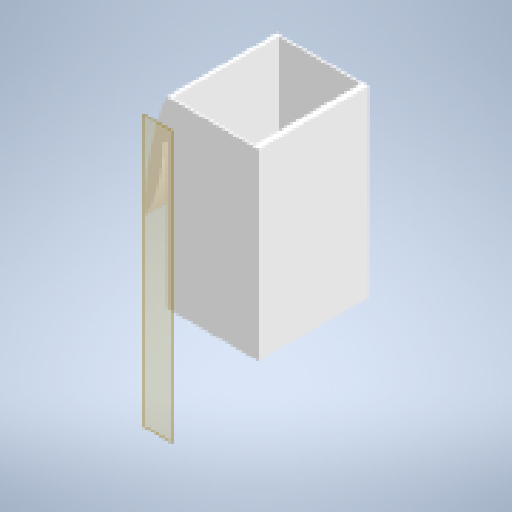
# Autodesk Inventor part: WingBox
Saved by Autodesk Inventor 2026 (Build 300175050, 175E)
## iProperties
Created: 2025-08-01
Part Number: WingBox
Material: Plastic, Opaque White
Document SubType Name: Modeling
Designer: Cupri
Mass: 728.648 g
Surface Area: 2482.51 cm^2
Volume: 765.387 cm^3
Density: 0.952 g/cm^3
Appearance: Smooth - White
Author: Cupri
Autodesk Inventor part; units mm, degrees
ref_plane "YZ Plane" through (0, 0, 0) normal (1, 0, 0) x (0, 1, 0)
ref_plane "XZ Plane" through (0, 0, 0) normal (0, 1, 0) x (-1, 0, 0)
ref_plane "XY Plane" through (0, 0, 0) normal (0, 0, 1) x (1, 0, 0)
ref_plane "Work Plane1" through (0, 0, 0) normal (0, 0, 1) x (1, 0, 0)
sketch "Sketch1" plane through (0, 0, 0) normal (0, 0, 1) x (1, 0, 0)
  line L0 (17.543857, 167.377737) -> (17.543857, -167.217661)
  line L1 (12.619782, 167.377737) -> (17.543857, 167.377737)
  arc A0 (12.619782, 167.377737) -> (7.619799, 162.364672) centre (12.619782, 162.377737) ccw
  arc A1 (-17.220572, 65.305302) -> (7.619799, 162.364672) centre (-192.379519, 161.842048) ccw
  spline S0 degree 3 poles (15.506608, -167.377737) (14.147951, -162.345779) (13.145398, -158.732995) (12.220923, -155.352167) (11.293739, -151.961434) (10.445107, -148.803984) (9.518675, -145.1939) (8.592185, -141.583591) (7.587911, -137.520736) (6.471828, -132.825116) (5.346807, -128.091892) (4.10798, -122.714929) (2.846807, -117.031098) (1.553707, -111.203383) (0.259478, -105.140337) (-0.92675, -99.276727) (-2.132162, -93.318284) (-3.225902, -87.566367) (-4.23784, -81.945311) (-5.5682, -74.555504) (-6.790359, -67.285613) (-7.971575, -59.836625) (-9.552302, -49.86823) (-11.026112, -39.596979) (-12.264211, -29.351416) (-13.140881, -22.09676) (-13.908596, -14.883997) (-14.596958, -7.852484) (-15.268141, -0.996451) (-15.867695, 5.674384) (-16.352254, 12.543674) (-16.713746, 17.668333) (-17.004603, 22.971721) (-17.201941, 28.510361) (-17.39909, 34.043661) (-17.502934, 39.811858) (-17.52457, 45.347495) (-17.543857, 50.282258) (-17.501315, 54.954248) (-17.410102, 59.083092) (-17.361094, 61.301547) (-17.298032, 63.363057) (-17.220572, 65.305302) knots 0 0 0 0 0.06599902 0.06599902 0.06599902 0.13219142 0.13219142 0.13219142 0.19838797 0.19838797 0.19838797 0.26511464 0.26511464 0.26511464 0.33353047 0.33353047 0.33353047 0.40305279 0.40305279 0.40305279 0.49445138 0.49445138 0.49445138 0.61676292 0.61676292 0.61676292 0.70336901 0.70336901 0.70336901 0.78781372 0.78781372 0.78781372 0.85081155 0.85081155 0.85081155 0.91374865 0.91374865 0.91374865 0.96985415 0.96985415 0.96985415 1 1 1 1
  line L2 (16.076195, -167.223946) -> (15.506608, -167.377737)
  line L3 (17.264865, -167.218855) -> (16.076195, -167.223946)
  line L4 (17.26486, -167.217661) -> (17.264865, -167.218855)
  line L5 (17.543857, -167.217661) -> (17.26486, -167.217661)
  line L6 (-7.380943, 65.327391) -> (-7.294185, 45.068724)
  line L7 (12.904649, 65.39642) -> (-7.380943, 65.327391)
  line L8 (12.973526, 45.15552) -> (12.904649, 65.39642)
  line L9 (-7.294185, 45.068724) -> (12.973526, 45.15552)
  arc A2 (12.543857, 221.029621) -> (-17.220572, 65.305302) centre (332.504822, 79.16708) ccw
  line L10 (12.543857, 221.029621) -> (17.543857, 221.029621)
  line L11 (17.543857, 221.029621) -> (17.543857, 167.377737)
  line L12 (17.543857, 167.377737) -> (12.619782, 167.377737)
  arc A3 (12.619782, 167.577737) -> (7.419799, 162.364149) centre (12.619782, 162.377737) ccw
  line L13 (12.619782, 167.577737) -> (17.743857, 167.577737)
  line L14 (17.743857, 167.577737) -> (17.743857, -167.417661)
  line L15 (17.743857, -167.417661) -> (17.544285, -167.417661)
  line L16 (17.544285, -167.417661) -> (16.103141, -167.423832)
  line L17 (16.103141, -167.423832) -> (15.365657, -167.622957)
  arc A4 (-17.41853, 65.360482) -> (7.419799, 162.364149) centre (-192.379519, 161.842048) ccw
  point P0 (0, 0)
  point P1 (-17.235714, 65.692749)
  point P2 (17.543857, 167.577737)
  dimension "d0" = 5
  dimension "d10" = 350
  dimension "d11" = 0.2
  constraints: 16 end point, 7 point on circle, 3 centre point, 2 parallel, 1 concentric, 1 horizontal, 1 perpendicular, 8 other
  measures "d0" distance of L10.start L10.end
  measures "d10" radius of A2
  measures "d11" radial gap between concentric circles of A1 A4
sketch "Sketch1 outline for Extrusion1" plane through (0, 0, 0) normal (0, 0, 1) x (1, 0, 0)
  line L0 (17.543857, 221.029621) -> (12.543857, 221.029621)
  line L1 (17.543857, 167.577737) -> (17.543857, 221.029621)
  line L2 (12.619782, 167.577737) -> (17.543857, 167.577737)
  arc A0 (7.419799, 162.364149) -> (12.619782, 167.577737) centre (12.619782, 162.377737) cw
  arc A1 (-17.235714, 65.692749) -> (7.419799, 162.364149) centre (-192.379519, 161.842048) ccw
  arc A2 (12.543857, 221.029621) -> (-17.235714, 65.692749) centre (332.504822, 79.16708) ccw
extrude "Extrusion1" add sketch "Sketch1 outline for Extrusion1" against normal blind 150
sketch "Sketch2" plane through (12.543857, 221.029621, 0) normal (0, 1, 0) x (1, 0, 0)
  line L0 (0.075924, 0) -> (-4.924076, 0)
  line L1 (0.075924, 0) -> (125.075924, 0)
  line L2 (125.075924, 0) -> (125.075924, 150)
  line L3 (125.075924, 150) -> (0.075924, 150)
  line L4 (0.075924, 150) -> (0.075924, 0)
  line L5 (5, 0) -> (5, 150)
  line L6 (5, 2.5) -> (117.075924, 2.5)
  line L7 (117.075924, 2.5) -> (117.075924, 147.5)
  line L8 (117.075924, 147.5) -> (5, 147.5)
  line L9 (5, 147.5) -> (5, 2.5)
  line L10 (5, 150) -> (10, 150)
  line L11 (10, 150) -> (10, 0)
  line L12 (10, 0) -> (5, 0)
  line L13 (5, 0) -> (5, 150)
  point P0 (-12.543857, 0)
  point P1 (-4.924059, 0)
  point P2 (5, 147.5)
  point P3 (10, 2.5)
  point P4 (10, 147.5)
  dimension "d3" = 125
  dimension "d4" = 2.5
  dimension "d5" = 2.5
  dimension "d6" = 8
  dimension "d9" = 5
  constraints: 24 end point, 6 parallel, 3 horizontal, 3 perpendicular, 2 point on line
  measures "d3" distance of L3.end L2.end
  measures "d4" distance between parallel lines of L1 L6
  measures "d5" distance between parallel lines of L3 L8
  measures "d6" distance between parallel lines of L2 L7
  measures "d9" distance of L11.end L12.end
extrude "Extrusion2" add sketch "Sketch2" against normal blind 250 contours L5 L6 L11 L1 | L11 L6 L7 L8 L3 L2 L1 | L5 L8 L11 L6 | L3 L11 L8 L5
body "Solid1"
